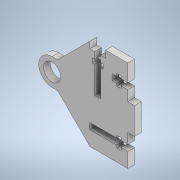
# Autodesk Inventor part: крепление оси
Saved by Autodesk Inventor 2020 (Build 240168000, 168)
## iProperties
Created: 2025-01-19
Part Number: крепление оси
Material: Типовые
Document SubType Name: Modeling
Designer: frozj
Density: 1 g/cm^3
Appearance: По умолчанию
Author: frozj
Autodesk Inventor part; units mm, degrees
ref_plane "YZ Plane" through (0, 0, 0) normal (1, 0, 0) x (0, 1, 0)
ref_plane "XZ Plane" through (0, 0, 0) normal (0, 1, 0) x (-1, 0, 0)
ref_plane "XY Plane" through (0, 0, 0) normal (0, 0, 1) x (1, 0, 0)
sketch "Эскиз1" plane through (0, 0, 0) normal (0, 0, 1) x (1, 0, 0)
  line L0 (10, -28.5) -> (-10, -28.5)
  line L1 (-10, -28.5) -> (-10, 28.5)
  line L2 (-10, 28.5) -> (10, 28.5)
  line L3 (10, 28.5) -> (10, -28.5)
  line L4 (10, -28.5) -> (-10, 28.5) construction
  line L5 (-10, -28.5) -> (10, 28.5) construction
  line L6 (-10, 28.5) -> (-27, 28.5)
  line L7 (-27, 28.5) -> (-27, -28.5)
  line L8 (-27, -28.5) -> (-10, -28.5)
  line L9 (-10, -28.5) -> (-10, 28.5)
  line L10 (-27, -28.5) -> (-27, 28.5)
  line L11 (10, 28.5) -> (-10, 28.5)
  line L12 (-10, 28.5) -> (-10, 25.5)
  line L13 (-10, 25.5) -> (10, 25.5)
  line L14 (10, 25.5) -> (10, 28.5)
  line L15 (10, 25.5) -> (7, 25.5)
  line L16 (7, 25.5) -> (7, -28.5)
  line L17 (7, -28.5) -> (10, -28.5)
  line L18 (10, -28.5) -> (10, 25.5)
  line L19 (7, 25.5) -> (-3, 25.5)
  line L20 (-3, 25.5) -> (-3, 28.5)
  line L21 (-3, 28.5) -> (7, 28.5)
  line L22 (7, 28.5) -> (7, 25.5)
  line L23 (-10, 25.5) -> (-3, 28.5)
  line L24 (-3, 25.5) -> (-10, 28.5)
  line L25 (-6.5, 27) -> (-6.5, 17)
  line L26 (7, 25.5) -> (10, 25.5)
  line L27 (10, 25.5) -> (10, 13.5)
  line L28 (10, 13.5) -> (7, 13.5)
  line L29 (7, 13.5) -> (7, 25.5)
  line L30 (7, 25.5) -> (10, 13.5)
  line L31 (7, 13.5) -> (10, 25.5)
  line L32 (8.5, 19.5) -> (0, 19.5)
  line L33 (-6.5, 27) -> (-5.15, 27)
  line L34 (-5.15, 27) -> (-5.15, 28.5)
  line L35 (-5.15, 28.5) -> (-6.5, 28.5)
  line L36 (-6.5, 28.5) -> (-6.5, 27)
  line L37 (-5.15, 28.5) -> (-7.85, 28.5)
  line L38 (-7.85, 28.5) -> (-7.85, 8.5)
  line L39 (-7.85, 8.5) -> (-5.15, 8.5)
  line L40 (-5.15, 8.5) -> (-5.15, 28.5)
  line L41 (-5.15, 25.5) -> (-4.05, 25.5)
  line L42 (-4.05, 25.5) -> (-4.05, 22.5)
  line L43 (-4.05, 22.5) -> (-5.15, 22.5)
  line L44 (-5.15, 22.5) -> (-5.15, 25.5)
  line L45 (-4.05, 22.5) -> (-8.95, 22.5)
  line L46 (-8.95, 22.5) -> (-8.95, 20.6)
  line L47 (-8.95, 20.6) -> (-4.05, 20.6)
  line L48 (-4.05, 20.6) -> (-4.05, 22.5)
  line L49 (8.5, 19.5) -> (10, 19.5)
  line L50 (10, 19.5) -> (10, 18.15)
  line L51 (10, 18.15) -> (8.5, 18.15)
  line L52 (8.5, 18.15) -> (8.5, 19.5)
  line L53 (10, 18.15) -> (0, 18.15)
  line L54 (0, 18.15) -> (0, 20.85)
  line L55 (0, 20.85) -> (10, 20.85)
  line L56 (10, 20.85) -> (10, 18.15)
  line L57 (7, 18.15) -> (4, 18.15)
  line L58 (4, 18.15) -> (4, 17.05)
  line L59 (4, 17.05) -> (7, 17.05)
  line L60 (7, 17.05) -> (7, 18.15)
  line L61 (4, 17.05) -> (2.1, 17.05)
  line L62 (2.1, 17.05) -> (2.1, 21.95)
  line L63 (2.1, 21.95) -> (4, 21.95)
  line L64 (4, 21.95) -> (4, 17.05)
  line L65 (7, 13.5) -> (10, 13.5)
  line L66 (10, 13.5) -> (10, 1.5)
  line L67 (10, 1.5) -> (7, 1.5)
  line L68 (7, 1.5) -> (7, 13.5)
  line L69 (7, 1.5) -> (10, 1.5)
  line L70 (10, 1.5) -> (10, -10.5)
  line L71 (10, -10.5) -> (7, -10.5)
  line L72 (7, -10.5) -> (7, 1.5)
  line L73 (8.5, 7.5) -> (7, 7.5)
  line L74 (10, -3.15) -> (0, -3.15)
  line L75 (0, -5.85) -> (10, -5.85)
  line L76 (4, -2.05) -> (2.1, -2.05)
  line L77 (2.1, -2.05) -> (2.1, -6.95)
  line L78 (2.1, -6.95) -> (4, -6.95)
  line L79 (4, -6.95) -> (4, -2.05)
  line L80 (0, -5.85) -> (-6, -5.85)
  line L81 (-6, -3.15) -> (0, -3.15)
  line L82 (0, -3.15) -> (0, -5.85)
  line L83 (10, -5.85) -> (-10, -5.85)
  line L84 (-10, -5.85) -> (-10, -3.15)
  line L85 (-10, -3.15) -> (10, -3.15)
  line L86 (10, -3.15) -> (10, -5.85)
  line L87 (-27, 28.5) -> (-27, 8)
  line L88 (-17.0714, 4) -> (0.879, 4) construction
  line L89 (-10, -12.4989) -> (10, -12.4989)
  circle A0 centre (-27, 8) radius 3.85
  line L90 (-27, 28.5) -> (-33, 28.5)
  line L91 (-33, 28.5) -> (-33, -28.5)
  line L92 (-33, -28.5) -> (-27, -28.5)
  line L93 (-27, -28.5) -> (-27, 28.5)
  circle A1 centre (-27, 8) radius 6
  line L94 (-10, 28.5) -> (-24.5, 14)
  line L95 (-10, 28.5) -> (10.5061, 28.5) construction
  line L96 (-24.5, 14) -> (-27, 14)
  line L97 (-10, -12.4989) -> (-24.5, 2.0011)
  line L98 (-10, -12.4989) -> (10.5061, -12.4989) construction
  line L99 (-24.5, 2.0011) -> (-27, 2)
  point P0 (0, 0)
  point P1 (2.1, 18.15)
  point P2 (2.1, 20.85)
  point P3 (4, 20.85)
  point P4 (7, 20.85)
  point P5 (7, 28.5)
  point P6 (-3, 25.5)
  point P7 (-5.15, 20.6)
  point P8 (-7.85, 20.6)
  point P9 (-7.85, 22.5)
  point P10 (-7.85, 25.5)
  point P11 (7, -5.85)
  point P12 (4, -5.85)
  point P13 (2.1, -5.85)
  point P14 (2.1, -3.15)
  point P15 (4, -3.15)
  point P16 (7, -3.15)
  point P17 (7, 18.15)
  point P18 (2.1, -5.85)
  point P19 (7, -5.85)
  point P20 (4, -5.85)
  point P21 (-10, -28.5)
  point P22 (-27, 12)
  point P23 (-27, 4)
  point P24 (7, -12.4989)
  dimension "d0" = 20
  dimension "d1" = 57
  dimension "d2" = 17
  dimension "d4" = 3
  dimension "d5" = 3
  dimension "d6" = 10
  dimension "d7" = 10
  dimension "d8" = 12
  dimension "d9" = 1.35
  dimension "d10" = 2.7
  dimension "d11" = 20
  dimension "d12" = 1.1
  dimension "d13" = 3
  dimension "d14" = 4.9
  dimension "d15" = 1.9
  dimension "d16" = 1.35
  dimension "d17" = 2.7
  dimension "d18" = 3
  dimension "d19" = 1.1
  dimension "d20" = 1.9
  dimension "d21" = 4.9
  dimension "d22" = 12
  dimension "d23" = 12
  dimension "d27" = 20
  dimension "d28" = 20.5
  dimension "d31" = 7.7
  dimension "d32" = 6
  dimension "d33" = 135
  dimension "d34" = 135
  constraints: 200 end point, 37 parallel, 23 horizontal, 20 perpendicular, 20 point on line, 8 symmetric about line, 5 midpoint, 2 centre point, 2 equal length, 2 point on circle, 1 coincident, 1 tangent
  measures "d0" distance of L1.end L2.end
  measures "d1" distance of L0.end L1.end
  measures "d2" distance of L8.end L7.end
  measures "d4" distance of L12.end L11.end
  measures "d5" distance of L17.end L16.end
  measures "d6" distance of L20.end L21.end
  measures "d7" distance of L25.start L25.end
  measures "d8" distance of L26.end L27.end
  measures "d9" distance of L35.end L34.end
  measures "d10" distance of L39.end L38.end
  measures "d11" distance of L38.end L37.end
  measures "d12" distance of L42.end L43.end
  measures "d13" distance of L41.end L42.end
  measures "d14" distance of L47.end L46.end
  measures "d15" distance of L46.end L45.end
  measures "d16" distance of L49.end L50.end
  measures "d17" distance of L53.end L54.end
  measures "d18" distance of L59.end L58.end
  measures "d19" distance of L58.end L57.end
  measures "d20" distance of L62.end L63.end
  measures "d21" distance of L61.end L62.end
  measures "d22" distance of L65.end L66.end
  measures "d23" distance of L69.end L70.end
  measures "d27" distance of L84.end L85.end
  measures "d28" distance of L6.end L87.end
  measures "d31" diameter of A0
  measures "d32" distance of L92.end L91.end
  measures "d33" angle of L94 L95
  measures "d34" angle of L98 L97
extrude "Выдавливание1" add sketch "Эскиз1" along normal blind 3 contours L7 A0 A1 | L89 L1 L83 L80 L75 L77 L78 L79 L16 | L97 L99 A1 L96 L94 L1 | L1 L13 L38 L45 L46 L47 L39 L40 L48 L42 L16 L55 L64 L63 L62 L54 L53 L61 L59 L74 L79 L76 L77 L81 L85 | L67 L16 L28 L3 | L59 L58 L53 L16 | L13 L42 L43 L40 | L2 L22 L13 L20
